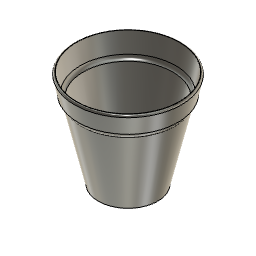
assembly (Autodesk Fusion 360 archive; units mm, degrees)
design "Vase"
Autodesk Fusion 360 part; units mm, degrees
sketch "Sketch1" plane through (0, 0, 0) normal (1, 0, 0) x (0, 1, 0)
  line L0 (0, 0) -> (0, 170)
  line L1 (0, 0) -> (50, 0)
  line L2 (0, 170) -> (92, 170)
  line L3 (92, 170) -> (84.0129, 130)
  line L4 (84.0129, 130) -> (80.0129, 130)
  line L5 (80.0129, 130) -> (50, 0)
  dimension "d1" = 170
  dimension "d2" = 50
  dimension "d4" = 92
  dimension "d5" = 40
  dimension "d6" = 4
  dimension "d7" = 103
  constraint coincident L0.start L1.start
  constraint vertical L0
  constraint perpendicular L0 L1
  constraint perpendicular L0 L2
  constraint parallel L2 L4
  measures "d1" distance of L0.start L0.end
  measures "d2" distance of L0.start L1.end
  measures "d4" distance of L0.end L2.end
  measures "d5" vertical distance of L2.end L3.end
  measures "d6" distance of L3.end L4.end
  measures "d7" angle of L1 L5
revolve "Revolve1" add sketch "Sketch1" angle 360 about axis through (0, 0, 0) along (0, 0, 1)
fillet "Fillet1" radius 10 1 edges at (-78.3275, 30.3803, 130)
shell "Shell1" thickness 4 outward yes removed faces 1 at (30.5809, -2.2917, 170)
fillet "Fillet2" radius 3 1 edges at (-34.7436, -89.577, 170)
fillet "Fillet3" radius 0.02 1 edges at (-85.7741, 33.2686, 170)
